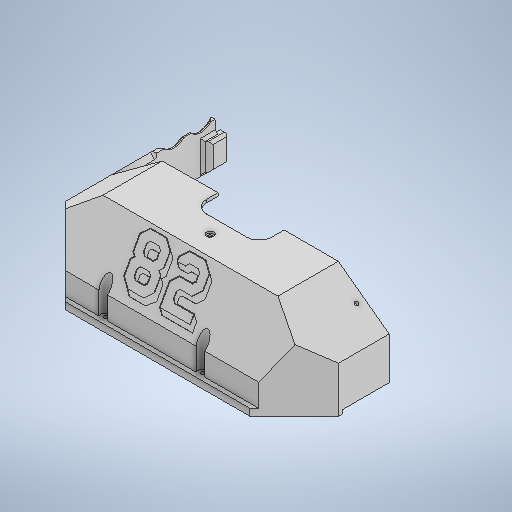
# Autodesk Inventor part: BackCover
Saved by Autodesk Inventor 2025.1 (Build 291241000, 241)
## iProperties
Created: 2026-04-16
Part Number: BackCover
Material: Generic
Document SubType Name: Modeling
Designer: User
Density: 1 g/cm^3
Appearance: Default
Author: User
## iProperties of the stored document BackCover_3DPrint.ipt
Created: 2026-04-16
Part Number: BackCover_3DPrint
Material: Generic
Document SubType Name: Modeling
Designer: User
Density: 1 g/cm^3
Appearance: Default
Author: User
Autodesk Inventor part; units mm, degrees
(part 1 of 2)
ref_plane "YZ Plane" through (0, 0, 0) normal (1, 0, 0) x (0, 1, 0)
ref_plane "XZ Plane" through (0, 0, 0) normal (0, 1, 0) x (-1, 0, 0)
ref_plane "XY Plane" through (0, 0, 0) normal (0, 0, 1) x (1, 0, 0)
sketch "Sketch1" plane through (0, 0, 0) normal (0, 0, 1) x (1, 0, 0)
  line L0 (39.244426, 3.5) -> (46, 3.5)
  line L1 (44, 0.5) -> (46, 3.5)
  line L2 (51, 0.5) -> (44, 0.5)
  line L3 (49, 3.5) -> (51, 0.5)
  line L4 (49, 3.5) -> (109.788954, 3.5)
  line L5 (107.788954, 0.5) -> (109.788954, 3.5)
  line L6 (114.788954, 0.5) -> (107.788954, 0.5)
  line L7 (112.788954, 3.5) -> (114.788954, 0.5)
  line L8 (112.788954, 3.5) -> (171, 3.5)
  line L9 (169, 0.5) -> (171, 3.5)
  line L10 (174, 3.5) -> (176, 0.5)
  line L11 (176, 0.5) -> (169, 0.5)
  line L12 (174, 3.5) -> (183.333482, 3.5)
  line L13 (183.333482, 3.713) -> (173.602006, 3.713)
  line L14 (173.602006, 3.713) -> (175.602006, 0.713)
  line L15 (175.602006, 0.713) -> (169.397994, 0.713)
  line L16 (169.397994, 0.713) -> (171.397994, 3.713)
  line L17 (171.397994, 3.713) -> (112.39096, 3.713)
  line L18 (112.39096, 3.713) -> (114.39096, 0.713)
  line L19 (114.39096, 0.713) -> (108.186948, 0.713)
  line L20 (108.186948, 0.713) -> (110.186948, 3.713)
  line L21 (110.186948, 3.713) -> (48.602006, 3.713)
  line L22 (48.602006, 3.713) -> (50.602006, 0.713)
  line L23 (50.602006, 0.713) -> (44.397994, 0.713)
  line L24 (44.397994, 0.713) -> (46.397994, 3.713)
  line L25 (46.397994, 3.713) -> (39.244426, 3.713)
  line L26 (39.244426, 3.713) -> (39.244426, 6.213)
  line L27 (39.244426, 3.713) -> (41.744426, 3.713) construction
  line L28 (39.244426, 6.213) -> (183.333482, 6.213)
  line L29 (183.333482, 6.213) -> (183.333482, 3.713)
  point P0 (0, 0)
  dimension "d0" = 0.213
  dimension "d1" = 2.5
  dimension "d2" = 90
  dimension "d3" = 90
  constraints: 34 end point, 2 perpendicular, 1 horizontal, 1 vertical, 12 other
  measures "d0" distance between parallel lines of L4 L21
  measures "d1" distance of L25.end L26.end
  measures "d2" angle of L27 L26
  measures "d3" angle of L26 L28
ref_plane "Work Plane1" through (44, 0.5, -3.5) normal (0, 0, 1) x (1, 0, 0)
extrude "Extrusion1" add sketch "Sketch1" against normal up to surface (3.5 mm away)
sketch "Sketch2" plane through (39.244426, 6.213, 0) normal (0, 1, 0) x (1, 0, 0)
  circle A0 centre (25.374082, 3) radius 1.5
  circle A1 centre (102.650051, 3) radius 1.5
  line L0 (144.089056, 0) -> (0, 0)
  circle A2 centre (25.374082, 3) radius 4
  circle A3 centre (102.650051, 3) radius 4
  point P0 (-39.244426, 0)
  point P1 (28.019834, 0)
  point P2 (22.728331, 0)
  point P3 (105.295802, 0)
  point P4 (100.004299, 0)
  dimension "d7" = 8
  dimension "d8" = 8
  constraints: 2 centre point, 2 coincident
  measures "d7" diameter of A2
  measures "d8" diameter of A3
extrude "Extrusion2" add sketch "Sketch2" against normal up to surface (2.5 mm away) contours L0 A3 | L0 A2 picked at (102.589783, 0.503646) picked at (25.313814, 0.503646)
sketch "Sketch3" plane through (39.244426, 6.213, 0) normal (0, 1, 0) x (1, 0, 0)
  arc A0 (26.788296, 3.5) -> (23.959869, 3.5) centre (25.374082, 3) ccw
  circle A1 centre (25.374082, 3) radius 1.5
  arc A2 (104.064264, 3.5) -> (101.235837, 3.5) centre (102.650051, 3) ccw
  circle A3 centre (102.650051, 3) radius 1.5
  point P0 (-39.244426, 0)
  point P1 (101.235837, 3.5)
  point P2 (104.064264, 3.5)
  constraints: 2 centre point, 2 coincident
extrude "Extrusion3" cut sketch "Sketch3" against normal blind 10
sketch "Sketch4" plane through (39.244426, 6.213, 0) normal (0, 1, 0) x (1, 0, 0)
  line L0 (144.089056, 0) -> (0, 0)
  line L1 (0, 0) -> (7.153568, 0)
  line L2 (0, 0) -> (144.089056, 0)
  line L3 (144.089056, 0) -> (144.089056, -2.5)
  line L4 (144.089056, -2.5) -> (0, -2.5)
  line L5 (0, -2.5) -> (0, 0)
  point P0 (-39.244426, 0)
  dimension "d13" = 2.5
  constraints: 8 end point, 2 parallel, 1 horizontal, 1 perpendicular
  measures "d13" distance of L2.end L3.end
extrude "Extrusion4" add sketch "Sketch4" against normal up to surface (5.5 mm away)
sketch "Sketch5" plane through (110.186948, 3.713, 0) normal (0, 0, -1) x (-1, 0, 0)
  line L0 (-63.415058, 0) -> (-73.146534, 0)
  line L1 (-73.146534, 0) -> (-73.146534, -3)
  line L2 (-73.146534, -3) -> (-65.415058, -3)
  line L3 (-65.415058, -3) -> (-63.415058, 0)
  line L4 (-61.211046, 0) -> (-59.211046, -3)
  line L5 (-59.211046, -3) -> (-4.204012, -3)
  line L6 (-4.204012, -3) -> (-2.204012, 0)
  line L7 (-2.204012, 0) -> (-61.211046, 0)
  line L8 (59.584942, -3) -> (61.584942, 0)
  line L9 (61.584942, 0) -> (0, 0)
  line L10 (2, -3) -> (59.584942, -3)
  line L11 (0, 0) -> (2, -3)
  line L12 (70.942522, 0) -> (63.788954, 0)
  line L13 (63.788954, 0) -> (65.788954, -3)
  line L14 (65.788954, -3) -> (70.942522, -3)
  line L15 (70.942522, 0) -> (70.942522, -3)
  point P0 (110.186948, -3.713)
extrude "Extrusion5" cut sketch "Sketch5" against normal blind 0.3
sketch "Sketch6" plane through (141.894477, 6.213, -3) normal (0, 1, 0) x (1, 0, 0)
  line L0 (-133.894477, 28.244426) -> (-102.650051, -3)
  line L1 (-134.106609, 28.032294) -> (-102.862183, -3.212132)
  line L2 (-102.650051, 0.5) -> (-102.650051, -5.5)
  line L3 (-125.61475, 19.540435) -> (-141.894477, 35.820162)
  line L4 (-102.862183, -3.212132) -> (-102.650051, -3.424264)
  line L5 (-102.650051, -5.5) -> (-141.894477, 33.744426)
  line L6 (-141.894477, 35.820162) -> (-141.894477, 33.744426)
  point P0 (-141.894477, -3)
  dimension "d18" = 0.3
  constraints: 10 end point, 4 point on line, 1 parallel, 1 vertical
  measures "d18" distance between parallel lines of L0 L1
extrude "Extrusion6" add sketch "Sketch6" against normal up to surface (5.5 mm away)
sketch "Sketch7" plane through (39.244426, 3.713, -3.5) normal (-1, 0, 0) x (0, 0, 1)
  line L0 (3.924264, -3) -> (3.924264, 2.5)
  line L1 (0, 2.5) -> (3.924264, 2.5)
  line L2 (0, 0) -> (0, 2.5)
  line L3 (0, 0) -> (3.8, 0)
  line L4 (3.8, 0) -> (3.8, -3)
  line L5 (3.8, -3) -> (3.924264, -3)
  point P0 (3.5, -3.713)
extrude "Extrusion7" add sketch "Sketch7" along normal up to surface surface through (0, 6.213, -38.820162) normal (0.7071068, 0, -0.7071068)
sketch "Sketch8" plane through (141.894477, 6.213, -3) normal (0, 1, 0) x (1, 0, 0)
  line L0 (41.439005, -3) -> (70.105523, 25.666518)
  line L1 (41.651137, -3.212132) -> (70.317655, 25.454386)
  line L2 (73.105523, 28.666518) -> (78.105523, 33.666518)
  line L3 (75.105523, 30.666518) -> (68.105523, 23.666518)
  line L4 (59.272099, 14.40883) -> (78.105523, 33.242254)
  line L5 (41.439005, -5.5) -> (41.439005, 0.5)
  line L6 (41.651137, -3.212132) -> (41.439005, -3.424264)
  line L7 (41.439005, -5.5) -> (78.105523, 31.166518)
  line L8 (78.105523, 31.166518) -> (78.105523, 33.242254)
  point P0 (-141.894477, -3)
  dimension "d23" = 0.3
  constraints: 10 end point, 3 point on line, 2 parallel, 1 vertical
  measures "d23" distance between parallel lines of L0 L1
extrude "Extrusion8" add sketch "Sketch8" against normal up to surface (5.5 mm away)
sketch "Sketch9" plane through (183.333482, 3.713, -3.5) normal (1, 0, 0) x (0, 0, -1)
  line L0 (-3.924264, 2.5) -> (-3.924264, -3)
  line L1 (-3.924264, -3) -> (-3.8, -3)
  line L2 (-3.8, -3) -> (-3.8, 0)
  line L3 (-3.8, 0) -> (0, 0)
  line L4 (0, 2.5) -> (0, 0)
  line L5 (-3.924264, 2.5) -> (0, 2.5)
  point P0 (-3.5, -3.713)
extrude "Extrusion9" add sketch "Sketch9" along normal up to surface surface through (183.333482, 6.213, 0.424264) normal (-0.7071068, 0, -0.7071068)
sketch "Sketch10" plane through (141.894477, 6.213, -3) normal (0, 1, 0) x (1, 0, 0)
  line L0 (78.105523, 33.242254) -> (45.363269, 0.5)
  line L1 (41.439005, -5.5) -> (78.105523, 31.166518)
  line L2 (42.146112, -6.207107) -> (78.81263, 30.459411)
  line L3 (41.439005, -5.5) -> (42.853218, -5.5)
  line L4 (78.105523, 31.166518) -> (78.105523, 29.752304)
  point P0 (-141.894477, -3)
  dimension "d28" = 1
  constraints: 6 end point, 2 point on line, 1 horizontal, 1 parallel, 1 perpendicular
  measures "d28" distance between parallel lines of L1 L2
extrude "Extrusion10" add sketch "Sketch10" against normal up to surface (5.5 mm away)
sketch "Sketch11" plane through (141.894477, 6.213, -3) normal (0, 1, 0) x (1, 0, 0)
  line L0 (-141.894477, 33.744426) -> (-102.650051, -5.5)
  line L1 (-142.601584, 33.03732) -> (-103.357158, -6.207107)
  line L2 (-102.650051, -5.5) -> (42.853218, -5.5)
  line L3 (-102.650051, -5.5) -> (-104.064264, -5.5)
  line L4 (-141.894477, 33.744426) -> (-141.894477, 32.330213)
  point P0 (-141.894477, -3)
  dimension "d31" = 1
  constraints: 6 end point, 2 point on line, 1 collinear, 1 parallel, 1 perpendicular
  measures "d31" distance between parallel lines of L0 L1
extrude "Extrusion11" add sketch "Sketch11" against normal up to surface (5.5 mm away)
sketch "Sketch12" plane through (184.747696, 0.713, 2.5) normal (0, 0, 1) x (1, 0, 0)
  line L0 (-181.747696, -0.213) -> (-179.747696, 2.787)
  line L1 (-174.747696, -0.213) -> (-181.747696, -0.213)
  line L2 (-176.747696, 2.787) -> (-174.747696, -0.213)
  line L3 (-184.747696, 2.787) -> (-179.747696, 2.787)
  line L4 (-176.747696, 2.787) -> (-145.503269, 2.787)
  line L5 (-184.747696, 3.018) -> (-179.337701, 3.018)
  line L6 (-179.337701, 3.018) -> (-181.349701, 0)
  line L7 (-184.747696, 0) -> (-146.917483, 0)
  line L8 (-175.14569, 0) -> (-177.15769, 3.018)
  line L9 (-177.15769, 3.018) -> (-173.551196, 3.018)
  line L10 (-184.747696, 5.5) -> (-184.747696, 0)
  line L11 (-184.747696, 5.5) -> (-146.917483, 5.5)
  line L12 (-173.551196, 3.018) -> (-173.551196, 5.5)
  point P0 (-184.747696, -0.713)
  constraints: 2 end point, 1 perpendicular, 1 point on line
extrude "Extrusion12" add sketch "Sketch12" against normal blind 76.008 contours L6 L5 L10 L11 L12 L9 L8 L7
sketch "Sketch13" plane through (141.894477, 6.213, -3) normal (0, 1, 0) x (1, 0, 0)
  line L0 (-130.697978, -5.5) -> (-130.697978, 21.133713)
  line L1 (-141.894477, 70.508) -> (-141.894477, -5.5)
  line L2 (-130.697978, -5.5) -> (-141.894477, -5.5)
  line L3 (-130.697978, 21.133713) -> (-104.064264, -5.5)
  line L4 (-141.894477, 32.330213) -> (-138.496483, 28.932219)
  line L5 (-130.697978, 21.133713) -> (-141.894477, 32.330213)
  point P0 (-141.894477, -3)
  constraints: 2 end point, 1 collinear
extrude "Extrusion13" cut sketch "Sketch13" against normal blind 76.008
sketch "Sketch14" plane through (184.747696, 0.713, 2.5) normal (0, 0, 1) x (1, 0, 0)
  line L0 (25.252304, -0.213) -> (27.252304, 2.787)
  line L1 (32.252304, -0.213) -> (25.252304, -0.213)
  line L2 (30.252304, 2.787) -> (32.252304, -0.213)
  line L3 (30.252304, 2.787) -> (35.252304, 2.787)
  line L4 (-1.414214, 2.787) -> (27.252304, 2.787)
  line L5 (-1.414214, 3) -> (27.650299, 3)
  line L6 (27.650299, 3) -> (25.650299, 0)
  line L7 (25.650299, 0) -> (31.85431, 0)
  line L8 (31.85431, 0) -> (29.85431, 3)
  line L9 (29.85431, 3) -> (35.252304, 3)
  line L10 (-184.747696, 5.5) -> (-173.551196, 5.5)
  line L11 (0, 5.5) -> (35.252304, 5.5)
  line L12 (35.252304, 5.5) -> (35.252304, 3)
  line L13 (35.252304, 5.5) -> (35.252304, 0)
  line L14 (35.252304, 5.5) -> (23.336304, 5.5)
  line L15 (23.336304, 5.5) -> (23.336304, 3)
  point P0 (-184.747696, -0.713)
  dimension "d38" = 0.213
  dimension "d39" = 11.1965
  dimension "d40" = 11.916
  constraints: 16 end point, 2 point on line, 1 collinear, 1 perpendicular, 4 other
  measures "d38" distance between parallel lines of L0 L6
  measures "d39" distance of L10.start L10.end
  measures "d40" distance of L11.end L14.end
extrude "Extrusion14" add sketch "Sketch14" against normal up to surface (76.008 mm away)
sketch "Sketch15" plane through (141.894477, 6.213, -3) normal (0, 1, 0) x (1, 0, 0)
  line L0 (42.853218, -5.5) -> (66.189523, 17.836304)
  line L1 (78.105523, -5.5) -> (78.105523, 70.508)
  line L2 (66.189523, -5.5) -> (66.189523, 17.836304)
  line L3 (78.105523, 29.752304) -> (72.707529, 24.35431)
  line L4 (66.189523, 17.836304) -> (78.105523, 29.752304)
  line L5 (78.105523, -5.5) -> (66.189523, -5.5)
  point P0 (-141.894477, -3)
  constraints: 2 end point, 1 collinear
extrude "Extrusion15" cut sketch "Sketch15" against normal blind 10
sketch "Sketch16" plane through (141.894477, 6.213, -3) normal (0, 1, 0) x (1, 0, 0)
  circle A0 centre (0, 0) radius 1.5
  circle A1 centre (-77.275968, 0) radius 1.5
  line L0 (-106.574315, 0.5) -> (-81.244595, 0.5)
  line L1 (-73.307341, 0.5) -> (-3.968627, 0.5)
  line L2 (3.968627, 0.5) -> (45.363269, 0.5)
  line L3 (3.968627, -2) -> (45.363269, -2)
  line L4 (-73.307341, -2) -> (-3.968627, -2)
  line L5 (-106.574315, -2) -> (-81.244595, -2)
  circle A2 centre (-77.275968, 0) radius 3.968627
  circle A3 centre (-77.275968, 0) radius 6.468627
  circle A4 centre (0, 0) radius 4
  line L6 (4, -2) -> (-3.968627, -2)
  line L7 (-73.307341, -2) -> (-81.244595, -2)
  circle A5 centre (0, 0) radius 6.5
  line L8 (-141.894477, 32.330213) -> (-104.064264, -5.5)
  line L9 (-106.574315, 0.5) -> (-130.697978, 24.623663)
  line L10 (42.853218, -5.5) -> (78.105523, 29.752304)
  line L11 (66.189523, 21.326254) -> (45.363269, 0.5)
  line L12 (40.66083, -2) -> (46.353218, -2)
  line L13 (-104.064264, 0.5) -> (-110.064264, 0.5)
  line L14 (-102.114502, -2) -> (-107.564264, -2)
  line L15 (45.363269, 0.5) -> (31.707529, 0.5)
  line L16 (40.08628, 0.5) -> (48.853218, 0.5)
  line L17 (42.853218, -5.5) -> (78.105523, 29.752304)
  point P0 (-141.894477, -3)
  point P1 (48.853218, 0.5)
  point P2 (6.480741, 0.5)
  point P3 (-6.480741, 0.5)
  point P4 (-70.826694, 0.5)
  point P5 (-83.725242, 0.5)
  point P6 (-110.064264, 0.5)
  point P7 (-80.703796, -2)
  point P8 (-73.848141, -2)
  point P9 (-3.464102, -2)
  point P10 (3.464102, -2)
  dimension "d45" = 2.5
  dimension "d46" = 2.5
  dimension "d47" = 2.5
  dimension "d48" = 2.5
  dimension "d49" = 2.5
  constraints: 18 end point, 10 point on line, 4 centre point, 3 parallel, 2 coincident, 2 horizontal
  measures "d45" distance between parallel lines of L2 L3
  measures "d46" distance between parallel lines of L1 L4
  measures "d47" distance between parallel lines of L0 L5
  measures "d48" radial gap between concentric circles of A2 A3
  measures "d49" radial gap between concentric circles of A4 A5
extrude "Extrusion16" add sketch "Sketch16" along normal blind 2.5 contours L0 A3 L5 L14 L8 L13 | A3 L4 L7 A2 L5 | L1 A5 L4 A3 | A5 L2 A4 L1 | L1 A4 L6 L4 A5 | A5 L3 L6 A4 L2 | L2 L16 L10 L12 L3 A5 picked at (-71.800275, 1.178196)
sketch "Sketch17" plane through (141.894477, 8.713, -3) normal (0, 1, 0) x (1, 0, 0)
  line L0 (48.853218, 0.5) -> (6.480741, 0.5)
  arc A0 (6.480741, 0.5) -> (-6.480741, 0.5) centre (0, 0) ccw
  line L1 (-6.480741, 0.5) -> (-70.826694, 0.5)
  arc A1 (-70.826694, 0.5) -> (-83.725242, 0.5) centre (-77.275968, 0) ccw
  line L2 (-83.725242, 0.5) -> (-110.064264, 0.5)
  line L3 (-110.064264, 0.5) -> (-107.564264, -2)
  line L4 (-107.564264, -2) -> (-80.703796, -2)
  arc A2 (-73.848141, -2) -> (-80.703796, -2) centre (-77.275968, 0) ccw
  line L5 (-73.848141, -2) -> (-3.464102, -2)
  arc A3 (3.464102, -2) -> (-3.464102, -2) centre (0, 0) ccw
  line L6 (3.464102, -2) -> (46.353218, -2)
  line L7 (46.353218, -2) -> (48.853218, 0.5)
  point P0 (-141.894477, -3)
ref_plane "Work Plane2" through (38.578251, 23.5, -49.929551) normal (0, 1, 0) x (0, 0, 1)
extrude "Extrusion17" add sketch "Sketch17" along normal up to surface (14.787 mm away)
sketch "Sketch18" plane through (0, 0.713, -35.330213) normal (-1, 0, 0) x (0, 0, 1)
  arc A0 (-38.129411, 114.141681) -> (-38.129411, 124.141641) centre (-51.274396, 119.141661) ccw
  line L0 (-6.468465, 53.643) -> (-6.468465, 43.143)
  line L1 (31.830213, 22.787) -> (8.876161, 63.893)
  line L2 (8.876161, 63.893) -> (-7.868465, 63.893)
  line L3 (25.830213, 22.787) -> (31.830213, 22.787)
  line L4 (31.830213, 22.787) -> (8.876161, 63.893)
  line L5 (-7.868465, 63.893) -> (-7.868465, 66.393)
  line L6 (-7.868465, 66.393) -> (10.343504, 66.393)
  line L7 (11.058902, 65.111868) -> (34.330213, 23.437723)
  line L8 (11.837038, 63.718387) -> (10.343504, 66.393)
  line L9 (34.330213, 22.787) -> (31.830213, 22.787)
  line L10 (34.330213, 22.787) -> (34.330213, 23.437723)
  point P0 (35.330213, -0.713)
  point P1 (11.058902, 65.111868)
  dimension "d63" = 2.5
  dimension "d64" = 90
  dimension "d65" = 2.5
  constraints: 16 end point, 2 point on circle, 2 point on line, 2 vertical, 1 centre point, 1 collinear, 1 parallel, 4 other
  measures "d63" distance of L2.end L5.end
  measures "d64" angle of L5 L6
  measures "d65" distance of L1.end L7.start
extrude "Extrusion20" add sketch "Sketch18" against normal up to surface (220 mm away)
sketch "Sketch20" plane through (50.602006, 0.713, 0.3) normal (0, -1, 0) x (1, 0, 0)
  line L0 (-50.602006, -35.630213) -> (-12.771793, 2.2)
  line L1 (-12.771793, 2.2) -> (134.14569, 2.2)
  line L2 (-50.602006, -35.630213) -> (-12.771793, -35.630213)
  line L3 (-12.771793, -35.630213) -> (-12.771793, 2.2)
  line L4 (-12.771793, 2.2) -> (-50.602006, 2.2)
  line L5 (-50.602006, 2.2) -> (-50.602006, -35.630213)
  point P0 (-50.602006, -0.3)
  constraints: 8 end point, 2 parallel, 1 horizontal, 1 perpendicular
extrude "Extrusion21" cut sketch "Sketch20" against normal through all contours L5 L4 L0
sketch "Sketch21" plane through (50.602006, 0.713, 0.3) normal (0, -1, 0) x (1, 0, 0)
  line L0 (134.14569, 2.2) -> (169.397994, -33.052304)
  line L1 (134.14569, 2.2) -> (169.397994, 2.2)
  line L2 (169.397994, 2.2) -> (169.397994, -33.052304)
  line L3 (169.397994, -33.052304) -> (134.14569, -33.052304)
  line L4 (134.14569, -33.052304) -> (134.14569, 2.2)
  point P0 (-50.602006, -0.3)
  constraints: 8 end point, 2 parallel, 1 horizontal, 1 perpendicular
extrude "Extrusion22" cut sketch "Sketch21" against normal through all contours L1 L2 L0
sketch "Sketch22" plane through (0, 67.106, -35.330213) normal (0, 1, 0) x (1, 0, 0)
  circle A0 centre (121.256446, 41.874226) radius 1.5
  circle A1 centre (121.256446, 65.148156) radius 1.5
  circle A2 centre (99.633064, 41.874226) radius 1.5
  circle A3 centre (99.633064, 65.148156) radius 1.5
  arc A4 (91.467089, 5.868465) -> (93.467089, 7.868465) centre (91.467089, 7.868465) ccw
  line L0 (91.467089, 5.868465) -> (77.45978, 5.868465)
  line L1 (77.45978, 5.868465) -> (77.45978, 2.868465)
  line L2 (143.95978, 2.868465) -> (77.45978, 2.868465)
  line L3 (143.95978, 2.868465) -> (143.95978, 5.868465)
  line L4 (143.95978, 5.868465) -> (138.25978, 5.868465)
  arc A5 (136.25978, 7.868465) -> (138.25978, 5.868465) centre (138.25978, 7.868465) ccw
  line L5 (136.25978, 7.868465) -> (136.25978, 31.682017)
  arc A6 (136.25978, 31.682017) -> (134.25978, 33.682017) centre (134.25978, 31.682017) ccw
  line L6 (134.25978, 33.682017) -> (128.659705, 33.682017)
  arc A7 (126.659705, 35.682017) -> (128.659705, 33.682017) centre (128.659705, 35.682017) ccw
  line L7 (126.659705, 35.682017) -> (126.659705, 49.382017)
  arc A8 (128.659705, 51.382017) -> (126.659705, 49.382017) centre (128.659705, 49.382017) ccw
  line L8 (128.659705, 51.382017) -> (134.25978, 51.382017)
  arc A9 (134.25978, 51.382017) -> (136.25978, 53.382017) centre (134.25978, 53.382017) ccw
  line L9 (136.25978, 53.382017) -> (136.25978, 91.068465)
  line L10 (136.25978, 91.068465) -> (141.95978, 91.068465)
  line L11 (141.95978, 91.068465) -> (141.95978, 94.068465)
  line L12 (141.95978, 94.068465) -> (132.95978, 94.068465)
  line L13 (132.95978, 94.068465) -> (132.95978, 86.768465)
  line L14 (126.95978, 80.768465) -> (132.95978, 86.768465)
  line L15 (126.95978, 80.768465) -> (124.60978, 80.768465)
  arc A10 (124.60978, 80.768465) -> (122.60978, 78.768465) centre (124.60978, 78.768465) ccw
  line L16 (122.60978, 78.768465) -> (122.60978, 74.568465)
  arc A11 (120.60978, 72.568465) -> (122.60978, 74.568465) centre (120.60978, 74.568465) ccw
  line L17 (120.60978, 72.568465) -> (99.30978, 72.568465)
  arc A12 (97.30978, 74.568465) -> (99.30978, 72.568465) centre (99.30978, 74.568465) ccw
  line L18 (97.30978, 74.568465) -> (97.30978, 78.768465)
  arc A13 (97.30978, 78.768465) -> (95.30978, 80.768465) centre (95.30978, 78.768465) ccw
  line L19 (95.30978, 80.768465) -> (92.95978, 80.768465)
  line L20 (86.95978, 86.768465) -> (92.95978, 80.768465)
  line L21 (86.95978, 86.768465) -> (86.95978, 94.068465)
  line L22 (86.95978, 94.068465) -> (77.95978, 94.068465)
  line L23 (77.95978, 94.068465) -> (77.95978, 91.068465)
  line L24 (77.95978, 91.068465) -> (85.456451, 91.068465)
  line L25 (85.456451, 91.068465) -> (85.456451, 85.968465)
  line L26 (85.456451, 85.968465) -> (84.65978, 85.968465)
  line L27 (84.65978, 85.968465) -> (84.65978, 61.175484)
  arc A14 (84.65978, 61.175484) -> (86.65978, 59.175484) centre (86.65978, 61.175484) ccw
  line L28 (86.65978, 59.175484) -> (92.229805, 59.175484)
  arc A15 (94.229805, 57.175484) -> (92.229805, 59.175484) centre (92.229805, 57.175484) ccw
  line L29 (94.229805, 57.175484) -> (94.229805, 36.174913)
  arc A16 (92.229805, 34.174913) -> (94.229805, 36.174913) centre (92.229805, 36.174913) ccw
  line L30 (92.229805, 34.174913) -> (86.65978, 34.174913)
  arc A17 (86.65978, 34.174913) -> (84.65978, 32.174913) centre (86.65978, 32.174913) ccw
  line L31 (84.65978, 32.174913) -> (84.65978, 24.481912)
  arc A18 (84.65978, 24.481912) -> (86.65978, 22.481912) centre (86.65978, 24.481912) ccw
  line L32 (86.65978, 22.481912) -> (91.467089, 22.481912)
  arc A19 (93.467089, 20.481912) -> (91.467089, 22.481912) centre (91.467089, 20.481912) ccw
  line L33 (93.467089, 20.481912) -> (93.467089, 7.868465)
  line L34 (98.70978, 20.347465) -> (98.70978, 18.397465)
  line L35 (121.56978, 36.132465) -> (121.56978, 17.852465)
  line L36 (98.70978, 36.132465) -> (98.70978, 17.852465)
  line L37 (98.70978, 17.852465) -> (121.56978, 17.852465)
  line L38 (110.13978, 17.852465) -> (110, 7.868465)
  line L39 (0, 7.868465) -> (220, 7.868465)
  line L40 (110, 7.868465) -> (109.929998, 2.868465)
  circle A20 centre (109.964999, 5.368465) radius 1.5
  circle A21 centre (109.964999, 5.368465) radius 1.5
  point P0 (0, -35.330213)
  dimension "d72" = 3
  constraints: 6 end point, 3 midpoint, 2 point on line, 1 centre point, 1 horizontal
  measures "d72" diameter of A20
extrude "Extrusion23" cut sketch "Sketch22" against normal blind 10 contours A20 L40 | L40 A20
sketch "Sketch23" plane through (0, 67.106, -35.330213) normal (0, 1, 0) x (1, 0, 0)
  circle A0 centre (109.964999, 5.368465) radius 1.5
  circle A1 centre (109.964999, 5.368465) radius 3
  point P0 (0, -35.330213)
  dimension "d75" = 6
  constraints: 1 centre point, 1 coincident
  measures "d75" diameter of A1
extrude "Extrusion24" cut sketch "Sketch23" against normal blind 1.5
sketch "Sketch24" plane through (31.830213, 6.213, -3.5) normal (0, 1, 0) x (1, 0, 0)
  line L0 (-31.830213, 70.008) -> (-31.830213, 31.830213)
  line L1 (-28.830213, 70.008) -> (-28.830213, 32.320162)
  line L2 (-31.830213, 31.830213) -> (0, 0)
  line L3 (3.489949, 0) -> (-20.633713, 24.123663)
  line L4 (0, 0) -> (3.489949, 0)
  line L5 (-7.033633, 10.523582) -> (-28.830213, 32.320162)
  line L6 (-31.830213, 70.008) -> (-20.633713, 70.008)
  point P0 (-31.830213, -3.5)
  dimension "d78" = 3
  constraints: 4 end point, 1 parallel, 1 point on line
  measures "d78" distance between parallel lines of L0 L1
extrude "Extrusion25" add sketch "Sketch24" along normal up to surface surface through (0, 23.5, -3.5) normal (0, -0.487547, -0.8730967)
sketch "Sketch25" plane through (10.343504, 67.106, -24.986709) normal (0, 1, 0) x (1, 0, 0)
  line L0 (-24.960228, 63.693537) -> (30.240364, 63.693537)
  line L1 (30.240364, 63.693537) -> (30.240364, -23.19024)
  line L2 (30.240364, -23.19024) -> (-24.960228, -23.19024)
  line L3 (-24.960228, -23.19024) -> (-24.960228, 63.693537)
  point P0 (-10.343504, -24.986709)
  constraints: 8 end point, 2 parallel, 1 horizontal, 1 perpendicular
extrude "Extrusion26" cut sketch "Sketch25" along normal through all
sketch "Sketch27" plane through (220, 67.106, -43.198678) normal (0, 0, -1) x (-1, 0, 0)
  line L0 (213.779028, -26.493702) -> (158.436266, 14.321511)
  line L1 (214.37257, -25.688899) -> (159.029807, 15.126315)
  line L2 (213.779028, -26.493702) -> (215.416407, -27.701267)
  line L3 (217.897382, -29.530983) -> (215.416407, -27.701267)
  line L4 (217.897382, -29.530983) -> (215.416407, -27.701267)
  line L5 (217.897382, -29.530983) -> (218.633638, -30.07397)
  line L6 (217.897382, -29.530983) -> (215.416407, -27.701267)
  line L7 (217.897382, -29.530983) -> (218.633638, -30.07397)
  line L8 (218.490924, -28.726179) -> (216.009948, -26.896464)
  line L9 (216.009948, -26.896464) -> (214.37257, -25.688899)
  line L10 (214.37257, -25.688899) -> (159.029807, 15.126315)
  line L11 (218.490924, -28.726179) -> (216.009948, -26.896464)
  line L12 (217, 0) -> (111.693313, 0)
  line L13 (220, 0) -> (217, 0)
  line L14 (220, -63.375) -> (220, 0)
  line L15 (179.540102, 0) -> (222.506281, -31.6875)
  point P0 (220, -67.106)
  point P1 (214.37257, -25.688899)
  point P2 (220, -29.839121)
extrude "Extrusion27" cut sketch "Sketch27" along normal through all both and the other way through all
sketch "Sketch28" plane through (0, 37.266879, -35.330213) normal (-0.5935415, 0.8048034, 0) x (0.8048034, 0.5935415, 0)
  line L0 (50.27302, 7.868465) -> (50.27302, -10.343504)
  line L1 (3.727618, 38.177787) -> (3.727618, 0.489949)
  line L2 (0, 0) -> (0, 38.177787)
  line L3 (50.27302, -10.343504) -> (50.27302, 38.177787)
  line L4 (50.27302, 38.177787) -> (0, 38.177787)
  line L5 (50.27302, -10.343504) -> (23.767794, -19.128402)
  line L6 (23.767794, -19.128402) -> (0, 0)
  point P0 (-22.119437, -35.330213)
  constraints: 4 end point, 1 perpendicular, 1 vertical
extrude "Extrusion28" add sketch "Sketch28" against normal blind 2.5
sketch "Sketch29" plane through (184.747696, 0.713, -73.508) normal (0, 0, -1) x (-1, 0, 0)
  line L0 (181.747696, 5.5) -> (181.747696, 35.660026)
  line L1 (184.747696, 27.791) -> (184.747696, 3.018)
  line L2 (184.747696, 3.018) -> (184.747696, 36.553879)
  line L3 (176.051196, 27.791) -> (176.051196, 5.518)
  line L4 (182.247696, 27.791) -> (176.051196, 27.791)
  line L5 (182.247696, 5.518) -> (182.247696, 27.791)
  line L6 (176.051196, 5.518) -> (182.247696, 5.518)
  line L7 (179.337701, 3.018) -> (184.747696, 3.018)
  line L8 (184.747696, 36.553879) -> (181.747696, 36.553879)
  line L9 (181.747696, 36.553879) -> (181.747696, 3.018)
  line L10 (181.747696, 3.018) -> (184.747696, 3.018)
  line L11 (184.747696, 3.018) -> (184.747696, 36.553879)
  line L12 (179.551196, 32.787) -> (179.551196, 30.787)
  line L13 (181.747696, 32.787) -> (184.747696, 32.787)
  line L14 (184.747696, 32.787) -> (184.747696, 3.018)
  line L15 (184.747696, 3.018) -> (181.747696, 3.018)
  line L16 (181.747696, 3.018) -> (181.747696, 32.787)
  point P0 (184.747696, -0.713)
  constraints: 16 end point, 4 parallel, 2 horizontal, 2 perpendicular, 2 point on line
ref_plane "Work Plane3" through (0, 0.713, -152.208182) normal (0, 0, 1) x (1, 0, 0)
extrude "Extrusion29" add sketch "Sketch29" along normal up to surface (78.700182 mm away) contours L13 L2 L1 L7 L9 L0 L6 L5 L4 | L4 L5 L6 L0
sketch "Sketch30" plane through (3, 33.5, -152.208182) normal (0, 0, -1) x (-1, 0, 0)
  line L0 (3, 0) -> (0, 0) projected
  line L1 (0, 0) -> (0, -29.769) projected
  line L2 (0, -29.769) -> (3, -29.769) projected
  line L3 (3, -29.769) -> (3, 0) projected
  point P0 (3, -33.5)
extrude "Extrusion30" cut sketch "Sketch30" against normal blind 0.5
sketch "Sketch31" plane through (3, 33.5, -151.708182) normal (0, 0, -1) x (-1, 0, 0)
  line L0 (-5.696499, -4.996) -> (-5.696499, -27.269)
  line L1 (0.5, -4.996) -> (-5.696499, -4.996)
  line L2 (0.5, -27.269) -> (0.5, -4.996)
  line L3 (-5.696499, -27.269) -> (0.5, -27.269)
  line L4 (-5.196499, -5.496) -> (-5.196499, -26.769)
  line L5 (-5.196499, -26.769) -> (0, -26.769)
  line L6 (0, -26.769) -> (0, -5.496)
  line L7 (0, -5.496) -> (-5.196499, -5.496)
  point P0 (3, -33.5)
  dimension "d98" = 0.5
  constraints: 8 end point, 3 other
  measures "d98" distance between parallel lines of L1 L7
extrude "Extrusion31" add sketch "Sketch31" along normal blind 5 contours L7 L6 L5 L4
sketch "Sketch32" plane through (3, 33.5, -151.708182) normal (0, 0, 1) x (1, 0, 0)
  line L0 (0, -5.496) -> (0, 0)
  line L1 (0, -29.769) -> (0, -26.769)
  line L2 (5.196499, -5.496) -> (5.196499, -26.769)
  line L3 (5.196499, -26.769) -> (0, -26.769)
  line L4 (0, -26.769) -> (0, -5.496)
  line L5 (5.196499, -26.769) -> (0, -26.769)
  line L6 (0, -26.769) -> (0, -5.496)
  line L7 (0, -5.496) -> (5.196499, -5.496)
  line L8 (5.196499, -5.496) -> (5.196499, -26.769)
  point P0 (-3, -33.5)
  constraints: 8 end point, 2 parallel, 1 horizontal, 1 perpendicular
extrude "Extrusion32" add sketch "Sketch32" along normal blind 10
chamfer "Chamfer1" distance 2 angle 45 5 edges at (8.1965, 28.004, -149.2082) (8.1965, 6.731, -149.2082) (3, 28.004, -146.7082) (3, 6.731, -146.7082) (3, 17.3675, -141.7082)
chamfer "Chamfer2" distance 3.1 angle 45 1 edges at (8.1965, 17.3675, -141.7082)
sketch "Sketch33" plane through (0, 37.266879, -35.330213) normal (-0.5935415, 0.8048034, 0) x (0.8048034, 0.5935415, 0)
  line L0 (0, 38.177787) -> (50.27302, 38.177787)
  line L1 (50.27302, 7.868465) -> (50.27302, 38.177787)
  line L2 (-2.235799, 38.177787) -> (0, 38.177787)
  line L3 (0, 0) -> (0, 38.177787)
  line L4 (50.27302, 38.177787) -> (0, 38.177787)
  line L5 (0, 38.177787) -> (0, 36.677787)
  line L6 (0, 36.677787) -> (50.27302, 36.677787)
  line L7 (50.27302, 36.677787) -> (50.27302, 38.177787)
  point P0 (-22.119437, -35.330213)
  point P1 (50.27302, 36.677787)
  dimension "d109" = 1.5
  constraints: 8 end point, 2 parallel, 1 horizontal, 1 perpendicular, 1 point on line
  measures "d109" distance of L5.end L4.end
extrude "Extrusion33" cut sketch "Sketch33" against normal blind 10
sketch "Sketch34" plane through (184.747696, 0.713, -73.508) normal (0, 0, -1) x (-1, 0, 0)
  line L0 (184.747696, 36.553879) -> (181.969627, 32.787)
  line L1 (181.969627, 32.787) -> (184.747696, 32.787)
  line L2 (184.747696, 32.787) -> (184.747696, 36.553879)
  line L3 (181.747696, 32.787) -> (181.969627, 32.787)
  line L4 (181.747696, 32.787) -> (181.747696, 32.486075)
  line L5 (181.747696, 32.787) -> (184.747696, 36.553879)
  point P0 (184.747696, -0.713)
  constraints: 2 end point
ref_plane "Work Plane4" through (5.196499, 33.7, -105.223419) normal (0, 0, 1) x (1, 0, 0)
extrude "Extrusion34" add sketch "Sketch34" along normal up to surface (31.715419 mm away)
sketch "Sketch35" plane through (3, 33.5, -105.223419) normal (0, 0, -1) x (-1, 0, 0)
  line L0 (3, 3.766879) -> (0, 0)
  line L1 (3, 0) -> (0, 0)
  line L2 (3, 0) -> (3, 3.766879)
  line L3 (0, 0) -> (3, 0)
  line L4 (3, 0) -> (3, 3.766879)
  line L5 (3, 3.766879) -> (0, 3.766879)
  line L6 (0, 3.766879) -> (0, 0)
  point P0 (3, -33.5)
  constraints: 8 end point, 2 parallel, 1 horizontal, 1 perpendicular
extrude "Extrusion35" add sketch "Sketch35" along normal up to surface (46.484763 mm away)
sketch "Sketch36" plane through (0, 0.713, -38.820162) normal (-1, 0, 0) x (0, 0, 1)
  circle A0 centre (-101.612165, 44.487) radius 8.8
  circle A1 centre (-79.953257, 44.487) radius 8.8
  circle A2 centre (-101.612165, 44.487) radius 11.3
  circle A3 centre (-79.953257, 44.487) radius 11.3
  point P0 (38.820162, -0.713)
  point P1 (-90.782711, 41.260094)
  point P2 (-90.782711, 47.713906)
  dimension "d116" = 2.5
  dimension "d117" = 2.5
  constraints: 2 centre point
  measures "d116" radial gap between concentric circles of A0 A2
  measures "d117" radial gap between concentric circles of A1 A3
extrude "Extrusion36" cut sketch "Sketch36" against normal blind 10 contours A0 | A1 | A2 A3 | A3 A2 picked at (-69.592471, 43.600194) picked at (-92.169663, 40.119365)
chamfer "Chamfer3" distance 2 angle 45 3 edges at (0, 33.9, -140.4323) (0, 33.9, -118.7734) (0, 37.2669, -129.6029)
chamfer "Chamfer4" distance 1 angle 45 4 edges at (4.5982, 6.731, -156.7082) (3, 17.3675, -156.7082) (4.5982, 28.004, -156.7082) (8.1965, 17.3675, -156.7082)
sketch "Sketch37" plane through (3, 33.199075, -73.508) normal (0, 0, 1) x (1, 0, 0)
  line L0 (-3, 4.067804) -> (0, 0)
  line L1 (0, 0.300925) -> (0, 0)
  line L2 (-3, 4.067804) -> (0, 0.300925)
  point P0 (-3, -33.199075)
extrude "Extrusion37" add sketch "Sketch37" along normal up to surface (1.5 mm away)
fillet "Fillet1" radius 2 2 edges at (1.5, 35.3834, -105.2234) (1.5, 35.3834, -72.008)
sketch "Sketch38" plane through (187.257746, 6.213, -3.5) normal (0, 1, 0) x (1, 0, 0)
  line L0 (3.489949, 0) -> (32.742254, 29.252304)
  line L1 (32.742254, 29.252304) -> (32.742254, 70.008)
  line L2 (30.242254, 70.008) -> (30.242254, 30.287838)
  line L3 (30.242254, 30.287838) -> (1.722183, 1.767767)
  line L4 (20.826254, 20.826254) -> (0, 0)
  line L5 (20.826254, 20.826254) -> (20.826254, 70.008)
  line L6 (0, 0) -> (3.489949, 0)
  line L7 (32.742254, 70.008) -> (20.826254, 70.008)
  point P0 (-187.257746, -3.5)
  point P1 (20.826254, 20.871838)
  dimension "d129" = 2.5
  constraints: 4 end point, 1 other
  measures "d129" distance between parallel lines of L1 L2
extrude "Extrusion38" add sketch "Sketch38" along normal up to surface contours L6 L4 L5 L3 L2 L7 L1 L0 surface through (0, 23.5, -3.5) normal (0, -0.487547, -0.8730967)
sketch "Sketch39" plane through (109.964999, 67.106, -40.698678) normal (0, 1, 0) x (1, 0, 0)
  line L0 (82.081549, 38.836854) -> (130.065798, 38.836854)
  line L1 (130.065798, 38.836854) -> (130.065798, -25.580354)
  line L2 (130.065798, -25.580354) -> (82.081549, -25.580354)
  line L3 (82.081549, -25.580354) -> (82.081549, 38.836854)
  point P0 (-109.964999, -40.698678)
  constraints: 8 end point, 2 parallel, 1 horizontal, 1 perpendicular
extrude "Extrusion39" cut sketch "Sketch39" along normal through all
sketch "Sketch40" plane through (37.830213, 6.213, 2.5) normal (0, 1, 0) x (1, 0, 0)
  arc A0 (30.216123, 3.5) -> (23.360469, 3.5) centre (26.788296, 5.5) ccw
  circle A1 centre (26.788296, 5.5) radius 1.5
  circle A2 centre (26.788296, 5.5) radius 3.968627
  circle A3 centre (104.064264, 5.5) radius 1.5
  arc A4 (108.032891, 6) -> (100.095637, 6) centre (104.064264, 5.5) ccw
  arc A5 (108.032891, 6) -> (100.095637, 6) centre (104.064264, 5.5) ccw
  circle A6 centre (104.064264, 5.5) radius 4
  point P0 (-37.830213, 2.5)
  constraints: 2 centre point, 2 coincident, 1 concentric
extrude "Extrusion40" cut sketch "Sketch40" along normal through all contours A2 A0 | A1 | A3 | A6 A4
sketch "Sketch41" plane through (64.618509, 23.5, -3) normal (0, 1, 0) x (1, 0, 0)
  line L0 (-6.449274, 0.5) -> (-3.937004, 0.5)
  arc A0 (3.937004, 0.5) -> (-3.937004, 0.5) centre (0, 0) ccw
  line L1 (3.937004, 0.5) -> (6.449274, 0.5)
  arc A1 (6.449274, 0.5) -> (-6.449274, 0.5) centre (0, 0) ccw
  point P0 (-64.618509, -3)
extrude "Extrusion41" add sketch "Sketch41" along normal up to surface surface through (0, 67.106, -24.986709) normal (0, 0.487547, 0.8730967)
sketch "Sketch42" plane through (141.894477, 23.5, -3) normal (0, 1, 0) x (1, 0, 0)
  line L0 (-6.480741, 0.5) -> (-3.968627, 0.5)
  arc A0 (3.968627, 0.5) -> (-3.968627, 0.5) centre (0, 0) ccw
  line L1 (3.968627, 0.5) -> (6.480741, 0.5)
  arc A1 (6.480741, 0.5) -> (-6.480741, 0.5) centre (0, 0) ccw
  point P0 (-141.894477, -3)
extrude "Extrusion42" add sketch "Sketch42" along normal up to surface surface through (0, 67.106, -24.986709) normal (0, 0.487547, 0.8730967)
sketch "Sketch43" plane through (141.894477, 6.213, -3) normal (0, -1, 0) x (1, 0, 0)
  arc A0 (-6.480741, -0.5) -> (6.480741, -0.5) centre (0, 0) ccw
  arc A1 (-3.968627, -0.5) -> (3.968627, -0.5) centre (0, 0) ccw
  line L0 (29.503517, -0.5) -> (3.968627, -0.5)
  line L1 (-3.968627, -0.5) -> (-29.503517, -0.5)
  arc A2 (-81.244595, -0.5) -> (-73.307341, -0.5) centre (-77.275968, 0) ccw
  arc A3 (-83.725242, -0.5) -> (-70.826694, -0.5) centre (-77.275968, 0) ccw
  line L2 (-31.707529, -0.5) -> (-73.307341, -0.5)
  line L3 (-81.244595, -0.5) -> (-93.292471, -0.5)
  point P0 (-141.894477, 3)
extrude "Extrusion43" add sketch "Sketch43" along normal up to surface (2.5 mm away)
chamfer "Chamfer5" distance 1 angle 45 9 edges at (141.8945, 3.713, -9.5) (159.8866, 3.713, -3.5) (180.4299, 3.713, -3.5) (123.9023, 3.713, -3.5) (90.6274, 3.713, -3.5) (64.6185, 3.713, -9.4686) (53.3856, 3.713, -3.5) (37.2823, 3.713, -3.5) (42.8212, 3.713, -3.5)
sketch "Sketch44" plane through (216.602006, 0.713, -73.508) normal (0, 0, -1) x (-1, 0, 0)
  line L0 (216.602006, 36.553879) -> (213.602006, 36.553879)
  line L1 (216.602006, 36.553879) -> (-3.397994, 36.553879)
  line L2 (-3.397994, 66.393) -> (-3.397994, 0)
  line L3 (216.602006, 36.553879) -> (436.602006, 36.553879) construction
  line L4 (-3.397994, 36.553879) -> (-0.891115, 36.553879)
  line L5 (176.142107, 66.393) -> (214.991291, 37.741779)
  line L6 (214.991291, 37.741779) -> (194.203196, 37.741779)
  line L7 (214.991291, 37.741779) -> (235.779386, 37.741779) construction
  line L8 (176.142107, 66.393) -> (4.367601, 66.393)
  line L9 (-3.397994, 36.553879) -> (33.012006, 36.553879) construction
  line L10 (-3.397994, 36.553879) -> (37.06002, 66.393)
  line L11 (-3.397994, 36.553879) -> (46.873509, 36.553879) construction
  line L12 (-1.914096, 34.541903) -> (38.543918, 64.381024)
  line L13 (175.319938, 63.893) -> (-0.897994, 63.893)
  line L14 (37.06002, 66.393) -> (38.543918, 64.381024)
  line L15 (-3.397994, 36.553879) -> (-1.914096, 34.541903)
  point P0 (216.602006, -0.713)
  dimension "d145" = 180
  dimension "d146" = 180
  dimension "d147" = 36.4087
  dimension "d150" = 36.41
  dimension "d151" = 2.5
  constraints: 22 end point, 4 horizontal, 3 equal length, 3 point on line, 2 parallel, 1 perpendicular
  measures "d145" angle of L1 L3
  measures "d146" angle of L6 L7
  measures "d147" angle of L6 L5
  measures "d150" angle of L11 L10
  measures "d151" distance between parallel lines of L10 L12
extrude "Extrusion44" add sketch "Sketch44" against normal up to surface surface through (0, 23.5, -3.5) normal (0, -0.487547, -0.8730967)
sketch "Sketch46" plane through (217.5, 39.110711, -33.787838) normal (0.5935594, 0.8047902, 0) x (0.8047902, -0.5935594, 0)
  line L0 (-65.02165, -53.334733) -> (22.283643, -53.334733)
  line L1 (22.283643, -53.334733) -> (22.283643, 58.076316)
  line L2 (22.283643, 58.076316) -> (-65.02165, 58.076316)
  line L3 (-65.02165, 58.076316) -> (-65.02165, -53.334733)
  point P0 (-151.827343, -33.787838)
  constraints: 8 end point, 2 parallel, 1 horizontal, 1 perpendicular
extrude "Extrusion45" cut sketch "Sketch46" along normal through all
sketch "Sketch47" plane through (50.602006, 0.713, 0.3) normal (0, -1, 0) x (1, 0, 0)
  line L0 (134.14569, 2.2) -> (169.397994, -33.052304)
  line L1 (169.397994, 2.170749) -> (134.14569, 2.170749)
  line L2 (134.14569, 2.170749) -> (134.14569, -33.052304)
  line L3 (134.14569, -33.052304) -> (169.397994, -33.052304)
  line L4 (169.397994, -33.052304) -> (169.397994, 2.170749)
  point P0 (-50.602006, -0.3)
  point P1 (134.174941, 2.170749)
  constraints: 8 end point, 2 parallel, 1 horizontal, 1 perpendicular
extrude "Extrusion46" cut sketch "Sketch47" against normal through all contours L1 L4 L0
sketch "Sketch48" plane through (109.964999, 67.106, -40.698678) normal (0, 1, 0) x (1, 0, 0)
  line L0 (36.494781, 0.6) -> (36.494781, 85.6)
  line L1 (-35.505219, 85.6) -> (-35.505219, 0.6)
  line L2 (69.576987, 32.809322) -> (69.576987, 2.5)
  line L3 (1.658312, 2.5) -> (69.576987, 2.5)
  line L4 (-69.505101, 2.5) -> (-1.658312, 2.5)
  line L5 (-1.658312, 2.5) -> (1.658312, 2.5)
  line L6 (-69.505101, 2.5) -> (-69.505101, 31.309322)
  line L7 (69.576987, -15.711969) -> (69.576987, 2.5)
  line L8 (1.658312, 2.5) -> (69.576987, 2.5)
  arc A0 (-1.658312, 2.5) -> (1.658312, 2.5) centre (0, 0) ccw
  line L9 (-69.505101, 2.5) -> (-1.658312, 2.5)
  line L10 (-69.505101, 2.5) -> (-69.505101, -15.711969)
  line L11 (-69.505101, -15.711969) -> (69.576987, -15.711969)
  circle A1 centre (0, 0) radius 1.5
  circle A2 centre (0, 0) radius 3
  line L12 (59.576987, 32.809322) -> (59.576987, 12.5)
  line L13 (36.494781, 12.5) -> (1.658312, 12.5)
  line L14 (1.658312, 12.5) -> (-1.658312, 12.5)
  line L15 (-1.658312, 12.5) -> (-25.505219, 12.5)
  line L16 (-59.505101, 12.5) -> (-59.505101, 31.309322)
  line L17 (-69.505101, 31.309322) -> (69.576987, 32.809322)
  line L18 (26.494781, 0.6) -> (26.494781, 2.5)
  line L19 (26.494781, 12.5) -> (26.494781, 85.6)
  line L20 (-25.505219, 85.6) -> (-25.505219, 12.5)
  line L21 (-25.505219, 2.5) -> (-25.505219, 0.6)
  point P0 (-109.964999, -40.698678)
  point P1 (26.494781, 32.34468)
  point P2 (-25.505219, 31.783861)
  point P3 (-1.658312, 2.5)
  point P4 (1.658312, 2.5)
  dimension "d160" = 10
  constraints: 20 end point, 4 parallel, 4 point on line, 1 centre point, 1 coincident
  measures "d160" distance between parallel lines of L4 L15
extrude "Extrusion47" add sketch "Sketch48" against normal blind 2.5 contours L3 A2 L4 L1 L17 L20 L15 L14 L13 L0 | L0 L17 L2 L3 | L13 L19 L17 L0 | L6 L17 L1 L4
sketch "Sketch49" plane through (0, 65.606, -35.330213) normal (0, 1, 0) x (1, 0, 0)
  circle A0 centre (109.964999, 5.368465) radius 3
  circle A1 centre (109.964999, 5.368465) radius 1.5
  point P0 (0, -35.330213)
extrude "Extrusion48" add sketch "Sketch49" against normal blind 1
fillet "Fillet2" radius 10 2 edges at (84.4598, 65.856, -53.1987) (136.4598, 65.856, -53.1987)
chamfer "Chamfer6" distance 3 angle 45 4 edges at (217.5, 6.213, -53.6479) (212.792, 6.213, -29.0798) (7.0982, 6.213, -31.7219) (3, 6.213, -54.6641)
sketch "Sketch50" plane through (220, 37.266879, -32.752304) normal (0.5935594, 0.8047902, 0) x (0.8047902, -0.5935594, 0)
  circle A0 centre (-24.226589, 33.755696) radius 1.5
  point P0 (-154.933742, -32.752304)
extrude "Extrusion49" cut sketch "Sketch50" against normal blind 3
sketch "Sketch51" plane through (216.602006, 0.713, -73.508) normal (0, 0, -1) x (-1, 0, 0)
  line L0 (37.06002, 66.393) -> (-3.397994, 36.553879)
  line L1 (-3.397994, 3) -> (-3.397994, 36.553879)
  line L2 (2, 3) -> (-3.397994, 3)
  line L3 (0, 0) -> (2, 3)
  line L4 (6.204012, 0) -> (0, 0)
  line L5 (4.204012, 3) -> (6.204012, 0)
  line L6 (8.518006, 3) -> (4.204012, 3)
  line L7 (8.518006, 5.5) -> (8.518006, 3)
  line L8 (2.102006, 5.5) -> (8.518006, 5.5)
  line L9 (-0.897994, 8.5) -> (2.102006, 5.5)
  line L10 (-0.897994, 8.5) -> (-0.897994, 35.291312)
  line L11 (-0.897994, 35.291312) -> (38.543918, 64.381024)
  line L12 (38.543918, 64.381024) -> (37.06002, 66.393)
  line L13 (37.88222, 63.893) -> (38.543918, 64.381024)
  line L14 (80.142226, 63.893) -> (37.88222, 63.893)
  line L15 (80.142226, 66.393) -> (80.142226, 63.893)
  line L16 (37.06002, 66.393) -> (80.142226, 66.393)
  line L17 (38.543918, 64.381024) -> (37.06002, 66.393)
  point P0 (216.602006, -0.713)
  point P1 (37.88222, 63.893)
extrude "Extrusion50" cut sketch "Sketch51" against normal blind 0.5